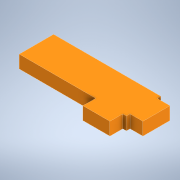
# Autodesk Inventor part: chassis_1_4
Saved by Autodesk Inventor 2022 (Build 260153000, 153)
## iProperties
Created: 2023-03-24
Part Number: chassis_1_4
Material: 一般
Document SubType Name: Modeling
Designer: Johnny Jou
Density: 79.16 g/cm^3
Appearance: 橙
Author: Johnny Jou
Autodesk Inventor part; units mm, degrees
ref_plane "YZ Plane" through (0, 0, 0) normal (1, 0, 0) x (0, 1, 0)
ref_plane "XZ Plane" through (0, 0, 0) normal (0, 1, 0) x (-1, 0, 0)
ref_plane "XY Plane" through (0, 0, 0) normal (0, 0, 1) x (1, 0, 0)
sketch "草圖5" plane through (0, 0, 0) normal (0, 1, 0) x (-1, 0, 0)
  line L0 (7.15, 3) -> (0.85, 3)
  line L1 (0.85, 3) -> (0.85, 0)
  line L2 (0.85, 0) -> (7.15, 0)
  line L3 (7.15, 0) -> (7.15, 3)
  line L4 (0, -0.85) -> (-3, -0.85)
  line L5 (-3, -0.85) -> (-3, -7.15)
  line L6 (-3, -7.15) -> (0, -7.15)
  line L7 (0, -7.15) -> (0, -0.85)
  line L8 (0, 0) -> (25, 0)
  line L9 (25, 0) -> (25, -8)
  line L10 (25, -8) -> (0, -8)
  line L11 (0, -8) -> (0, 0)
  point P0 (7.15, 0)
  dimension "d17" = 0.85
  dimension "d18" = 0.85
  dimension "d19" = 3
  dimension "d20" = 6.3
  dimension "d21" = 6.3
  dimension "d22" = 25
  dimension "d23" = 8
  dimension "d24" = 3
  constraints: 24 end point, 6 parallel, 3 horizontal, 3 perpendicular, 2 collinear, 1 coincident
  measures "d17" distance between parallel lines of L8 L4
  measures "d18" distance between parallel lines of L11 L1
  measures "d19" distance between parallel lines of L2 L0
  measures "d20" distance of L0.start L0.end
  measures "d21" distance of L4.end L5.end
  measures "d22" distance of L9.end L10.end
  measures "d23" distance of L8.end L9.end
  measures "d24" distance between parallel lines of L7 L5
extrude "擠出3" add sketch "草圖5" along normal blind 3
equation "\"d18\" = d17"
equation "\"d20\" = d21"
